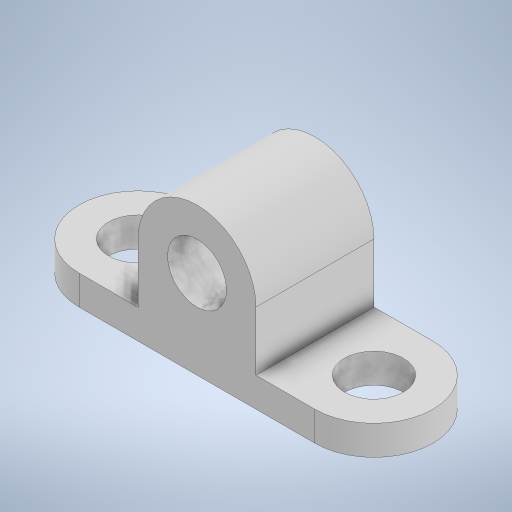
# Autodesk Inventor part: Actividad 1 Lab Dinámica Alison Martínez 1190119
Saved by Autodesk Inventor 2024 (Build 280153000, 153)
## iProperties
Created: 2024-02-07
Part Number: Actividad 1 Lab Dinámica Alison Martínez 1190119
Material: Genérico
Document SubType Name: Modeling
Designer: Alison
Density: 1 g/cm^3
Appearance: Valor por defecto
Author: Alison
Autodesk Inventor part; units mm, degrees
ref_plane "YZ Plane" through (0, 0, 0) normal (1, 0, 0) x (0, 1, 0)
ref_plane "XZ Plane" through (0, 0, 0) normal (0, 1, 0) x (-1, 0, 0)
ref_plane "XY Plane" through (0, 0, 0) normal (0, 0, 1) x (1, 0, 0)
sketch "Boceto2" plane through (0, 0, 0) normal (0, 0, 1) x (1, 0, 0)
  line L0 (20, -15) -> (-20, -15)
  line L1 (-20, -15) -> (-20, 15)
  line L2 (-20, 15) -> (20, 15)
  line L3 (20, 15) -> (20, -15)
  line L4 (20, -15) -> (-20, 15) construction
  line L5 (-20, -15) -> (20, 15) construction
  point P0 (0, 0)
  dimension "d7" = 40
  dimension "d8" = 30
  constraints: 12 end point, 2 midpoint, 2 parallel, 1 horizontal, 1 perpendicular
  measures "d7" distance of L1.end L2.end
  measures "d8" distance of L0.start L2.end
extrude "Extrusión2" add sketch "Boceto2" along normal blind 40
sketch "Boceto4" plane through (0, 0, 40) normal (0, 0, 1) x (1, 0, 0)
  line L0 (20, 15) -> (-20, 15) projected
  circle A0 centre (0, 15) radius 20
  point P0 (0, 0)
  constraints: 1 midpoint, 3 other
extrude "Extrusión3" add sketch "Boceto4" against normal blind 40 contours L0 A0 picked at (4.9901, 19.4208)
sketch "Boceto6" plane through (0, 0, 0) normal (0, 0, -1) x (-1, 0, 0)
  line L0 (-20, -15) -> (-20, 15) projected
  line L1 (-20, -15) -> (-40, -15)
  line L2 (-40, -15) -> (-40, -5)
  line L3 (-40, -5) -> (-20, -5)
  line L4 (-20, -5) -> (-20, -15)
  point P0 (0, 0)
  point P1 (-20, -5)
  dimension "d17" = 20
  dimension "d18" = 10
  constraints: 8 end point, 2 parallel, 1 horizontal, 1 perpendicular
  measures "d17" distance of L2.end L3.end
  measures "d18" distance of L1.end L2.end
extrude "Extrusión5" add sketch "Boceto6" against normal blind 40
sketch "Boceto7" plane through (0, 0, 0) normal (0, 0, -1) x (-1, 0, 0)
  line L0 (20, 15) -> (20, -15) projected
  line L1 (20, -15) -> (40, -15)
  line L2 (40, -15) -> (40, -5)
  line L3 (40, -5) -> (20, -5)
  line L4 (20, -5) -> (20, -15)
  point P0 (0, 0)
  dimension "d21" = 20
  dimension "d22" = 10
  constraints: 8 end point, 2 parallel, 1 horizontal, 1 perpendicular
  measures "d21" distance of L3.end L2.end
  measures "d22" distance of L2.end L1.end
extrude "Extrusión6" add sketch "Boceto7" against normal blind 40
sketch "Boceto8" plane through (-40, -5, 0) normal (0, 1, 0) x (1, 0, 0)
  circle A0 centre (0, -20) radius 20
  point P0 (40, 0)
  point P1 (0, 0)
  constraints: 1 vertical alignment, 2 other
extrude "Extrusión7" add sketch "Boceto8" against normal blind 10
sketch "Boceto9" plane through (20, -5, 0) normal (0, 1, 0) x (1, 0, 0)
  line L0 (20, 0) -> (-60, 0) projected
  line L1 (20, 0) -> (20, -40) projected
  circle A0 centre (20, -20) radius 20
  point P0 (-20, 0)
  point P1 (20, -40)
  constraints: 3 other
extrude "Extrusión8" add sketch "Boceto9" against normal blind 10 contours A0 L1 picked at (27.983, -21.6506)
sketch "Boceto10" plane through (0, 0, 0) normal (0, 0, -1) x (-1, 0, 0)
  arc A0 (20, 15) -> (-20, 15) centre (0, 15) ccw projected
  circle A1 centre (0, 15) radius 10
  point P0 (0, 0)
  dimension "d31" = 20
  constraints: 1 centre point, 1 coincident
  measures "d31" diameter of A1
extrude "Extrusión9" cut sketch "Boceto10" against normal blind 40
sketch "Boceto11" plane through (-20, -5, 40) normal (0, 1, 0) x (1, 0, 0)
  arc A0 (-20, 40) -> (-20, 0) centre (-20, 20) ccw projected
  circle A1 centre (-20, 20) radius 10
  point P0 (20, 40)
  dimension "d34" = 20
  constraints: 1 centre point, 1 coincident
  measures "d34" diameter of A1
extrude "Extrusión10" cut sketch "Boceto11" against normal blind 10
sketch "Boceto12" plane through (20, -5, 40) normal (0, 1, 0) x (1, 0, 0)
  arc A0 (20, 0) -> (20, 40) centre (20, 20) ccw projected
  circle A1 centre (20, 20) radius 10
  point P0 (-20, 40)
  dimension "d37" = 20
  constraints: 1 centre point, 1 coincident, 1 point on circle
  measures "d37" diameter of A1
extrude "Extrusión11" cut sketch "Boceto12" against normal blind 10
